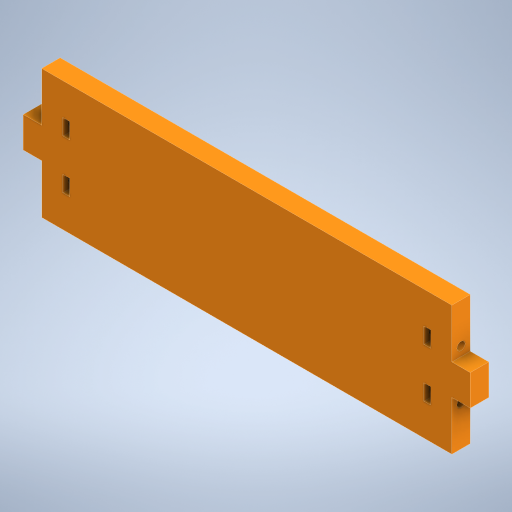
# Autodesk Inventor part: frame_upper3
Saved by Autodesk Inventor 2024 (Build 280153000, 153)
## iProperties
Created: 2024-09-08
Part Number: frame_upper3
Material: 일반
Document SubType Name: Modeling
Designer: jmha0
Density: 1 g/cm^3
Appearance: 주황색
Author: jmha0
Autodesk Inventor part; units mm, degrees
ref_plane "YZ Plane" through (0, 0, 0) normal (1, 0, 0) x (0, 1, 0)
ref_plane "XZ Plane" through (0, 0, 0) normal (0, 1, 0) x (-1, 0, 0)
ref_plane "XY Plane" through (0, 0, 0) normal (0, 0, 1) x (1, 0, 0)
sketch "스케치1" plane through (0, 0, 0) normal (0, 0, 1) x (1, 0, 0)
  line L0 (0, 0) -> (133.5, 0)
  line L1 (133.5, 0) -> (133.5, 42)
  line L2 (133.5, 42) -> (0, 42)
  line L3 (0, 42) -> (0, 0)
  dimension "d0" = 133.5
  dimension "d1" = 42
  constraints: 8 end point, 2 parallel, 1 horizontal, 1 perpendicular
  measures "d0" distance of L2.end L1.end
  measures "d1" distance of L1.end L0.end
extrude "돌출1" add sketch "스케치1" along normal blind 6
sketch "스케치2" plane through (133.5, 0, 0) normal (1, 0, 0) x (0, 0, -1)
  line L0 (0, 0) -> (0, 42) projected
  line L1 (0, 42) -> (-6, 42) projected
  line L2 (-6, 0) -> (-6, 42) projected
  line L3 (0, 0) -> (-6, 0) projected
  line L4 (-6, 16) -> (0, 16)
  line L5 (0, 16) -> (0, 26)
  line L6 (0, 26) -> (-6, 26)
  line L7 (-6, 26) -> (-6, 16)
  line L8 (-6, 16) -> (0, 26) construction
  line L9 (0, 16) -> (-6, 26) construction
  point P0 (-3, 21)
  dimension "d4" = 10
  constraints: 12 end point, 2 midpoint, 2 parallel, 1 horizontal, 1 perpendicular, 1 point on line
  measures "d4" distance of L5.end L4.end
extrude "돌출2" add sketch "스케치2" along normal blind 6 contours L4 L2 L6 L0
sketch "스케치3" plane through (0, 0, 0) normal (-1, 0, 0) x (0, 0, 1)
  line L0 (6, 26) -> (0, 26) projected
  line L1 (0, 16) -> (6, 16) projected
  line L2 (0, 42) -> (0, 0) projected
  line L3 (0, 0) -> (6, 0) projected
  line L4 (6, 42) -> (6, 0) projected
  line L5 (0, 42) -> (6, 42) projected
extrude "돌출3" add sketch "스케치3" along normal blind 6 contours L4 L1 L2 L0
sketch "스케치4" plane through (0, 42, 0) normal (-1, 0, 0) x (0, 0, 1)
  line L0 (0, -16) -> (6, -16) projected
  line L1 (6, 0) -> (6, -16) projected
  line L2 (0, 0) -> (6, 0) projected
  line L3 (0, 0) -> (0, -16) projected
  line L4 (6, -26) -> (0, -26) projected
  line L5 (0, -26) -> (0, -42) projected
  line L6 (0, -42) -> (6, -42) projected
  line L7 (6, -26) -> (6, -42) projected
  line L8 (0, -16) -> (6, -16)
  line L9 (6, -16) -> (6, -10)
  line L10 (6, -10) -> (0, -10)
  line L11 (0, -10) -> (0, -16)
  line L12 (6, -26) -> (0, -26)
  line L13 (0, -26) -> (0, -32)
  line L14 (0, -32) -> (6, -32)
  line L15 (6, -32) -> (6, -26)
  circle A0 centre (3, -13) radius 1.35
  circle A1 centre (3, -29) radius 1.35
  dimension "d9" = 6
  dimension "d10" = 6
  dimension "d11" = 6
  dimension "d12" = 6
  dimension "d13" = 2.7
  dimension "d14" = 2.7
  constraints: 16 end point, 4 parallel, 2 centre point, 2 horizontal, 2 perpendicular
  measures "d9" distance of L10.end L9.end
  measures "d10" distance of L9.end L8.end
  measures "d11" distance of L14.end L13.end
  measures "d12" distance of L13.end L12.end
  measures "d13" diameter of A0
  measures "d14" diameter of A1
extrude "돌출4" cut sketch "스케치4" against normal blind 16 contours A0 | A1
sketch "스케치5" plane through (133.5, 42, 6) normal (1, 0, 0) x (0, 0, -1)
  circle A0 centre (3, -13) radius 1.35 projected
  circle A1 centre (3, -29) radius 1.35 projected
  point P0 (6, -42)
extrude "돌출5" cut sketch "스케치5" against normal blind 16
sketch "스케치7" plane through (0, 0, 0) normal (0, 0, -1) x (-1, 0, 0)
  line L0 (-133.5, 0) -> (-133.5, 16) projected
  line L1 (-133.5, 11.65) -> (-133.5, 14.35) projected
  line L2 (-133.5, 0) -> (-133.5, 16) projected
  line L3 (-133.5, 11.65) -> (-133.5, 14.35) projected
  line L4 (-133.5, 0) -> (-133.5, 16) projected
  line L5 (-133.5, 0) -> (-133.5, 16) projected
  line L6 (-133.5, 42) -> (0, 42) projected
  line L7 (-133.5, 42) -> (0, 42) projected
  line L8 (0, 0) -> (-133.5, 0) projected
  line L9 (0, 0) -> (-133.5, 0) projected
  line L10 (-133.5, 16) -> (-139.5, 16) projected
  line L11 (-133.5, 16) -> (-139.5, 16) projected
  line L12 (-133.5, 16) -> (-139.5, 16) projected
  line L13 (-133.5, 16) -> (-139.5, 16) projected
  line L14 (-117.5, 11.65) -> (-117.5, 14.35) projected
  line L15 (-117.5, 11.65) -> (-117.5, 14.35) projected
  line L16 (-133.5, 11.65) -> (-133.5, 14.35) projected
  line L17 (-117.5, 11.65) -> (-117.5, 14.35) projected
  line L18 (-133.5, 26) -> (-139.5, 26) projected
  line L19 (-133.5, 26) -> (-139.5, 26) projected
  line L20 (-133.5, 26) -> (-139.5, 26) projected
  line L21 (-133.5, 26) -> (-139.5, 26) projected
  line L22 (-139.5, 26) -> (-139.5, 16) projected
  line L23 (-139.5, 16) -> (-139.5, 26) projected
  line L24 (-117.5, 27.65) -> (-117.5, 30.35) projected
  line L25 (-133.5, 27.65) -> (-133.5, 30.35) projected
  line L26 (-133.5, 26) -> (-133.5, 42) projected
  line L27 (-133.5, 26) -> (-133.5, 42) projected
  line L28 (-133.5, 27.65) -> (-133.5, 30.35) projected
  line L29 (-133.5, 26) -> (-133.5, 42) projected
  line L30 (-133.5, 26) -> (-133.5, 42) projected
  line L31 (0, 16) -> (0, 0) projected
  line L32 (0, 16) -> (0, 0) projected
  line L33 (0, 0) -> (-133.5, 0) projected
  line L34 (0, 0) -> (-133.5, 0) projected
  line L35 (-133.5, 0) -> (-133.5, 16) projected
  line L36 (-133.5, 16) -> (-139.5, 16) projected
  line L37 (-139.5, 26) -> (-139.5, 16) projected
  line L38 (-133.5, 26) -> (-139.5, 26) projected
  line L39 (-133.5, 26) -> (-133.5, 42) projected
  line L40 (-133.5, 42) -> (0, 42) projected
  line L41 (0, 42) -> (0, 26) projected
  line L42 (0, 26) -> (6, 26) projected
  line L43 (6, 16) -> (6, 26) projected
  line L44 (0, 16) -> (6, 16) projected
  line L45 (0, 16) -> (0, 0) projected
  line L46 (0, 0) -> (-133.5, 0) projected
  line L47 (-133.5, 0) -> (-133.5, 16) projected
  line L48 (0, 0) -> (-133.5, 0) projected
  line L49 (0, 16) -> (0, 0) projected
  line L50 (0, 16) -> (6, 16) projected
  line L51 (6, 26) -> (6, 16) projected
  line L52 (0, 26) -> (6, 26) projected
  line L53 (0, 42) -> (0, 26) projected
  line L54 (-133.5, 42) -> (0, 42) projected
  line L55 (-133.5, 26) -> (-133.5, 42) projected
  line L56 (-133.5, 26) -> (-139.5, 26) projected
  line L57 (-139.5, 16) -> (-139.5, 26) projected
  line L58 (-133.5, 16) -> (-139.5, 16) projected
  line L59 (0, 42) -> (0, 26) projected
  line L60 (0, 42) -> (0, 26) projected
  line L61 (-133.5, 42) -> (0, 42) projected
  line L62 (-133.5, 42) -> (0, 42) projected
  line L63 (-133.5, 27.65) -> (-133.5, 30.35) projected
  line L64 (-139.5, 26) -> (-139.5, 16) projected
  line L65 (-139.5, 16) -> (-139.5, 26) projected
  line L66 (-16, 14.35) -> (-16, 11.65) projected
  line L67 (-16, 14.35) -> (-16, 11.65) projected
  line L68 (0, 14.35) -> (0, 11.65) projected
  line L69 (0, 16) -> (0, 0) projected
  line L70 (0, 16) -> (0, 0) projected
  line L71 (-16, 30.35) -> (-16, 27.65) projected
  line L72 (0, 30.35) -> (0, 27.65) projected
  line L73 (-16, 14.35) -> (-16, 11.65) projected
  line L74 (0, 14.35) -> (0, 11.65) projected
  line L75 (0, 14.35) -> (0, 11.65) projected
  line L76 (0, 30.35) -> (0, 27.65) projected
  line L77 (0, 30.35) -> (0, 27.65) projected
  line L78 (0, 42) -> (0, 26) projected
  line L79 (0, 42) -> (0, 26) projected
  line L80 (6, 16) -> (6, 26) projected
  line L81 (0, 16) -> (6, 16) projected
  line L82 (6, 26) -> (6, 16) projected
  line L83 (6, 16) -> (6, 26) projected
  line L84 (0, 16) -> (6, 16) projected
  line L85 (0, 16) -> (6, 16) projected
  line L86 (0, 16) -> (6, 16) projected
  line L87 (0, 26) -> (6, 26) projected
  line L88 (0, 26) -> (6, 26) projected
  line L89 (0, 26) -> (6, 26) projected
  line L90 (6, 26) -> (6, 16) projected
  line L91 (-16, 30.35) -> (-16, 27.65) projected
  line L92 (-16, 30.35) -> (-16, 27.65) projected
  line L93 (0, 26) -> (6, 26) projected
  line L94 (-117.5, 27.65) -> (-117.5, 30.35) projected
  line L95 (-117.5, 27.65) -> (-117.5, 30.35) projected
  line L96 (-133.5, 30.35) -> (-117.5, 30.35) projected
  line L97 (-133.5, 27.65) -> (-117.5, 27.65) projected
  line L98 (-133.5, 14.35) -> (-117.5, 14.35) projected
  line L99 (-133.5, 11.65) -> (-117.5, 11.65) projected
  line L100 (0, 30.35) -> (-16, 30.35) projected
  line L101 (0, 27.65) -> (-16, 27.65) projected
  line L102 (0, 14.35) -> (-16, 14.35) projected
  line L103 (0, 11.65) -> (-16, 11.65) projected
  line L104 (-126.6, 26.4) -> (-124.4, 26.4)
  line L105 (-124.4, 26.4) -> (-124.4, 31.6)
  line L106 (-124.4, 31.6) -> (-126.6, 31.6)
  line L107 (-126.6, 31.6) -> (-126.6, 26.4)
  line L108 (-126.6, 26.4) -> (-124.4, 31.6) construction
  line L109 (-124.4, 26.4) -> (-126.6, 31.6) construction
  line L110 (-126.6, 10.4) -> (-124.4, 10.4)
  line L111 (-124.4, 10.4) -> (-124.4, 15.6)
  line L112 (-124.4, 15.6) -> (-126.6, 15.6)
  line L113 (-126.6, 15.6) -> (-126.6, 10.4)
  line L114 (-126.6, 10.4) -> (-124.4, 15.6) construction
  line L115 (-124.4, 10.4) -> (-126.6, 15.6) construction
  line L116 (-9.1, 26.4) -> (-6.9, 26.4)
  line L117 (-6.9, 26.4) -> (-6.9, 31.6)
  line L118 (-6.9, 31.6) -> (-9.1, 31.6)
  line L119 (-9.1, 31.6) -> (-9.1, 26.4)
  line L120 (-9.1, 26.4) -> (-6.9, 31.6) construction
  line L121 (-6.9, 26.4) -> (-9.1, 31.6) construction
  line L122 (-9.1, 10.4) -> (-6.9, 10.4)
  line L123 (-6.9, 10.4) -> (-6.9, 15.6)
  line L124 (-6.9, 15.6) -> (-9.1, 15.6)
  line L125 (-9.1, 15.6) -> (-9.1, 10.4)
  line L126 (-9.1, 10.4) -> (-6.9, 15.6) construction
  line L127 (-6.9, 10.4) -> (-9.1, 15.6) construction
  point P0 (-125.5, 29)
  point P1 (-125.5, 13)
  point P2 (-8, 29)
  point P3 (-8, 13)
  dimension "d27" = 2.2
  dimension "d28" = 5.2
  dimension "d29" = 5.2
  dimension "d30" = 2.2
  dimension "d31" = 5.2
  dimension "d32" = 5.2
  constraints: 48 end point, 8 midpoint, 8 parallel, 4 horizontal, 4 perpendicular, 2 point on line, 5 other
  measures "d27" distance of L106.end L105.end
  measures "d28" distance of L105.end L104.end
  measures "d29" distance of L111.end L110.end
  measures "d30" distance of L118.end L117.end
  measures "d31" distance of L117.end L116.end
  measures "d32" distance of L123.end L122.end
extrude "돌출7" cut sketch "스케치7" against normal blind 16 contours L113 L98 L111 L99 | L99 L111 L110 L113 | L113 L112 L111 L98 | L123 L122 L125 L103 | L103 L125 L102 L123 | L102 L125 L124 L123 | L107 L96 L105 L97 | L97 L105 L104 L107 | L107 L106 L105 L96 | L117 L116 L119 L101 | L101 L119 L100 L117 | L100 L119 L118 L117
sketch "스케치8" plane through (0, 0, 6) normal (0, 0, 1) x (1, 0, 0)
  line L0 (9.1, 26.4) -> (6.9, 26.4) projected
  line L1 (6.9, 26.4) -> (6.9, 31.6) projected
  line L2 (6.9, 31.6) -> (9.1, 31.6) projected
  line L3 (9.1, 31.6) -> (9.1, 26.4) projected
  line L4 (126.6, 10.4) -> (124.4, 10.4) projected
  line L5 (124.4, 10.4) -> (124.4, 15.6) projected
  line L6 (124.4, 15.6) -> (126.6, 15.6) projected
  line L7 (126.6, 15.6) -> (126.6, 10.4) projected
  line L8 (9.1, 10.4) -> (6.9, 10.4) projected
  line L9 (6.9, 10.4) -> (6.9, 15.6) projected
  line L10 (6.9, 15.6) -> (9.1, 15.6) projected
  line L11 (9.1, 15.6) -> (9.1, 10.4) projected
  line L12 (126.6, 26.4) -> (124.4, 26.4) projected
  line L13 (124.4, 26.4) -> (124.4, 31.6) projected
  line L14 (124.4, 31.6) -> (126.6, 31.6) projected
  line L15 (126.6, 31.6) -> (126.6, 26.4) projected
  line L16 (133.5, 0) -> (133.5, 16) projected
  line L17 (133.5, 16) -> (139.5, 16) projected
  line L18 (139.5, 26) -> (139.5, 16) projected
  line L19 (133.5, 26) -> (139.5, 26) projected
  line L20 (133.5, 26) -> (133.5, 42) projected
  line L21 (133.5, 42) -> (0, 42) projected
  line L22 (0, 42) -> (0, 26) projected
  line L23 (0, 26) -> (-6, 26) projected
  line L24 (-6, 16) -> (-6, 26) projected
  line L25 (0, 16) -> (-6, 16) projected
  line L26 (0, 16) -> (0, 0) projected
  line L27 (0, 0) -> (133.5, 0) projected
  line L28 (133.5, 0) -> (0, 0)
  line L29 (0, 0) -> (0, 42)
  line L30 (0, 42) -> (133.5, 42)
  line L31 (133.5, 42) -> (133.5, 0)
  constraints: 8 end point, 2 parallel, 1 horizontal, 1 perpendicular
extrude "돌출8" cut sketch "스케치8" against normal through all contours L31 L19 L18 L17 | L25 L24 L23 L29
sketch "스케치9" plane through (133.5, 0, 0) normal (1, 0, 0) x (0, 0, -1)
  circle A0 centre (-3, 29) radius 1.35 projected
  circle A1 centre (-3, 13) radius 1.35 projected
  line L0 (-6, 0) -> (-6, 42) projected
  line L1 (0, 0) -> (-6, 0) projected
  line L2 (0, 0) -> (0, 42) projected
  line L3 (0, 42) -> (-6, 42) projected
  line L4 (-6, 16) -> (0, 16)
  line L5 (0, 16) -> (0, 26)
  line L6 (0, 26) -> (-6, 26)
  line L7 (-6, 26) -> (-6, 16)
  line L8 (-6, 16) -> (0, 26) construction
  line L9 (0, 16) -> (-6, 26) construction
  point P0 (-3, 21)
  dimension "d37" = 10
  constraints: 12 end point, 2 midpoint, 2 parallel, 1 horizontal, 1 perpendicular, 1 point on line
  measures "d37" distance of L5.end L4.end
extrude "돌출9" add sketch "스케치9" along normal blind 6 contours L0 L6 L2 L4
sketch "스케치10" plane through (0, 0, 0) normal (-1, 0, 0) x (0, 0, 1)
  line L0 (6, 15.6) -> (6, 10.4) projected
  line L1 (6, 10.4) -> (6, 15.6) projected
  line L2 (0, 15.6) -> (0, 10.4) projected
  line L3 (6, 31.6) -> (6, 26.4) projected
  line L4 (0, 26.4) -> (0, 31.6) projected
  line L5 (0, 10.4) -> (0, 15.6) projected
  line L6 (6, 0) -> (6, 16) projected
  line L7 (0, 0) -> (0, 16) projected
  line L8 (0, 0) -> (6, 0) projected
  line L9 (0, 16) -> (6, 16) projected
  line L10 (6, 0) -> (6, 16) projected
  line L11 (0, 0) -> (6, 0) projected
  line L12 (0, 0) -> (0, 16) projected
  circle A0 centre (3, 13) radius 1.35 projected
  line L13 (6, 26) -> (6, 42) projected
  line L14 (0, 42) -> (6, 42) projected
  line L15 (6, 26) -> (0, 26) projected
  line L16 (0, 26) -> (0, 42) projected
  line L17 (0, 42) -> (6, 42) projected
  line L18 (6, 26) -> (6, 42) projected
  circle A1 centre (3, 29) radius 1.35 projected
  line L19 (0, 26) -> (0, 42) projected
  line L20 (0, 31.6) -> (0, 26.4) projected
  line L21 (6, 26.4) -> (6, 31.6) projected
  line L22 (6, 31.6) -> (6, 26.4) projected
  line L23 (6, 26.4) -> (6, 31.6) projected
  circle A2 centre (3, 29) radius 1.35 projected
  circle A3 centre (3, 29) radius 1.35 projected
  circle A4 centre (3, 13) radius 1.35 projected
  circle A5 centre (3, 13) radius 1.35 projected
  circle A6 centre (3, 29) radius 1.35 projected
  line L24 (0, 31.6) -> (6, 31.6) projected
  line L25 (0, 26.4) -> (6, 26.4) projected
  line L26 (6, 31.6) -> (6, 26.4) projected
  line L27 (0, 31.6) -> (6, 31.6) projected
  line L28 (0, 26.4) -> (0, 31.6) projected
  line L29 (0, 26.4) -> (6, 26.4) projected
  circle A7 centre (3, 29) radius 1.35 projected
  circle A8 centre (3, 29) radius 1.35 projected
  circle A9 centre (3, 29) radius 1.35 projected
  circle A10 centre (3, 13) radius 1.35 projected
  circle A11 centre (3, 13) radius 1.35 projected
  line L30 (0, 31.6) -> (6, 31.6) projected
  line L31 (0, 31.6) -> (6, 31.6) projected
  line L32 (0, 31.6) -> (6, 31.6) projected
  circle A12 centre (3, 29) radius 1.35 projected
  line L33 (0, 26.4) -> (6, 26.4) projected
  line L34 (6, 26.4) -> (6, 31.6) projected
  line L35 (0, 26.4) -> (6, 26.4) projected
  line L36 (0, 31.6) -> (0, 26.4) projected
  line L37 (0, 31.6) -> (6, 31.6) projected
  circle A13 centre (3, 29) radius 1.35 projected
  line L38 (0, 26.4) -> (6, 26.4) projected
  line L39 (0, 26.4) -> (6, 26.4) projected
  line L40 (0, 31.6) -> (0, 26.4) projected
  line L41 (0, 26.4) -> (0, 31.6) projected
  line L42 (6, 15.6) -> (6, 10.4) projected
  line L43 (0, 42) -> (6, 42) projected
  line L44 (0, 42) -> (6, 42) projected
  line L45 (6, 0) -> (6, 16) projected
  line L46 (6, 26) -> (6, 16) projected
  line L47 (6, 26) -> (6, 42) projected
  line L48 (6, 42) -> (6, 0) projected
  line L49 (6, 26.4) -> (6, 31.6) projected
  line L50 (6, 31.6) -> (6, 26.4) projected
  line L51 (6, 10.4) -> (6, 15.6) projected
  line L52 (6, 15.6) -> (6, 10.4) projected
  line L53 (6, 10.4) -> (6, 15.6) projected
  line L54 (6, 15.6) -> (6, 10.4) projected
  line L55 (6, 26.4) -> (6, 31.6) projected
  line L56 (6, 31.6) -> (6, 26.4) projected
  line L57 (0, 0) -> (0, 16) projected
  line L58 (0, 42) -> (0, 0) projected
  line L59 (0, 26) -> (0, 42) projected
  line L60 (0, 16) -> (0, 26) projected
  line L61 (0, 26.4) -> (0, 31.6) projected
  line L62 (0, 31.6) -> (0, 26.4) projected
  line L63 (0, 10.4) -> (0, 15.6) projected
  line L64 (0, 15.6) -> (0, 10.4) projected
  line L65 (0, 10.4) -> (0, 15.6) projected
  line L66 (0, 15.6) -> (0, 10.4) projected
  line L67 (0, 26.4) -> (0, 31.6) projected
  line L68 (0, 31.6) -> (0, 26.4) projected
  line L69 (0, 0) -> (6, 0) projected
  line L70 (0, 0) -> (6, 0) projected
  line L71 (0, 10.4) -> (0, 15.6) projected
  line L72 (0, 15.6) -> (0, 10.4) projected
  line L73 (6, 10.4) -> (6, 15.6) projected
  line L74 (6, 42) -> (6, 0) projected
  circle A14 centre (3, 29) radius 1.35 projected
  circle A15 centre (3, 13) radius 1.35 projected
  line L75 (0, 16) -> (0, 26) projected
  line L76 (6, 26) -> (6, 16) projected
  line L77 (6, 16) -> (0, 16) projected
  line L78 (0, 16) -> (6, 16) projected
  line L79 (0, 26) -> (6, 26) projected
  line L80 (6, 26) -> (0, 26) projected
  line L81 (6, 26) -> (6, 16) projected
  line L82 (6, 16) -> (0, 16) projected
  line L83 (0, 16) -> (0, 26) projected
  line L84 (0, 26) -> (6, 26) projected
  line L85 (0, 16) -> (6, 16) projected
  line L86 (6, 16) -> (0, 16) projected
  line L87 (6, 26) -> (0, 26) projected
  line L88 (0, 26) -> (6, 26) projected
  circle A16 centre (3, 29) radius 1.35 projected
  line L89 (0, 31.6) -> (6, 31.6) projected
  line L90 (0, 31.6) -> (6, 31.6) projected
  circle A17 centre (3, 29) radius 1.35 projected
  line L91 (0, 26.4) -> (6, 26.4) projected
  line L92 (0, 15.6) -> (6, 15.6) projected
  line L93 (0, 26.4) -> (6, 26.4) projected
  circle A18 centre (3, 13) radius 1.35 projected
  circle A19 centre (3, 13) radius 1.35 projected
  line L94 (0, 15.6) -> (6, 15.6) projected
  line L95 (0, 10.4) -> (6, 10.4) projected
  line L96 (0, 10.4) -> (6, 10.4) projected
  circle A20 centre (3, 13) radius 1.35 projected
  line L97 (0, 15.6) -> (6, 15.6) projected
  line L98 (0, 15.6) -> (6, 15.6) projected
  circle A21 centre (3, 13) radius 1.35 projected
  line L99 (0, 10.4) -> (6, 10.4) projected
  line L100 (0, 10.4) -> (6, 10.4) projected
  line L101 (6, 10.4) -> (6, 15.6) projected
  line L102 (0, 10.4) -> (6, 10.4) projected
  line L103 (0, 15.6) -> (0, 10.4) projected
  line L104 (0, 15.6) -> (6, 15.6) projected
  circle A22 centre (3, 13) radius 1.35 projected
  line L105 (0, 15.6) -> (6, 15.6) projected
  line L106 (0, 15.6) -> (6, 15.6) projected
  line L107 (6, 15.6) -> (6, 10.4) projected
  line L108 (0, 15.6) -> (6, 15.6) projected
  line L109 (0, 10.4) -> (0, 15.6) projected
  line L110 (0, 10.4) -> (6, 10.4) projected
  circle A23 centre (3, 13) radius 1.35 projected
  line L111 (0, 0) -> (6, 0) projected
  line L112 (0, 42) -> (0, 0) projected
  circle A24 centre (3, 13) radius 1.35 projected
  circle A25 centre (3, 29) radius 1.35 projected
  line L113 (6, 42) -> (6, 0) projected
  line L114 (0, 42) -> (6, 42) projected
  line L115 (0, 42) -> (0, 0) projected
  line L116 (0, 0) -> (6, 0) projected
  circle A26 centre (3, 13) radius 1.35 projected
  circle A27 centre (3, 29) radius 1.35 projected
  circle A28 centre (3, 13) radius 1.35 projected
  circle A29 centre (3, 13) radius 1.35 projected
  circle A30 centre (3, 13) radius 1.35 projected
  line L117 (0, 42) -> (6, 42) projected
  circle A31 centre (3, 29) radius 1.35 projected
  circle A32 centre (3, 29) radius 1.35 projected
  circle A33 centre (3, 29) radius 1.35 projected
  circle A34 centre (3, 13) radius 1.35 projected
  circle A35 centre (3, 29) radius 1.35 projected
  circle A36 centre (3, 13) radius 1.35 projected
  circle A37 centre (3, 13) radius 1.35 projected
  circle A38 centre (3, 29) radius 1.35 projected
  circle A39 centre (3, 29) radius 1.35 projected
  line L118 (6, 10.4) -> (6, 15.6) projected
  line L119 (0, 10.4) -> (6, 10.4) projected
  line L120 (0, 15.6) -> (0, 10.4) projected
  line L121 (0, 15.6) -> (6, 15.6) projected
  circle A40 centre (3, 13) radius 1.35 projected
  line L122 (6, 26.4) -> (6, 31.6) projected
  line L123 (0, 26.4) -> (6, 26.4) projected
  line L124 (0, 31.6) -> (0, 26.4) projected
  line L125 (0, 31.6) -> (6, 31.6) projected
  circle A41 centre (3, 29) radius 1.35 projected
  line L126 (0, 10.4) -> (6, 10.4) projected
  line L127 (0, 10.4) -> (6, 10.4) projected
  line L128 (0, 15.6) -> (6, 15.6) projected
  line L129 (0, 15.6) -> (6, 15.6) projected
  line L130 (0, 26.4) -> (6, 26.4) projected
  line L131 (0, 26.4) -> (6, 26.4) projected
  line L132 (0, 31.6) -> (6, 31.6) projected
  line L133 (0, 31.6) -> (6, 31.6) projected
  line L134 (6, 15.6) -> (6, 10.4) projected
  line L135 (0, 15.6) -> (6, 15.6) projected
  line L136 (0, 10.4) -> (0, 15.6) projected
  line L137 (0, 10.4) -> (6, 10.4) projected
  circle A42 centre (3, 13) radius 1.35 projected
  circle A43 centre (3, 29) radius 1.35 projected
  circle A44 centre (3, 29) radius 1.35 projected
  circle A45 centre (3, 13) radius 1.35 projected
  circle A46 centre (3, 13) radius 1.35 projected
  line L138 (6, 31.6) -> (6, 26.4) projected
  line L139 (0, 31.6) -> (6, 31.6) projected
  line L140 (0, 26.4) -> (0, 31.6) projected
  line L141 (0, 26.4) -> (6, 26.4) projected
  circle A47 centre (3, 29) radius 1.35 projected
  line L142 (0, 10.4) -> (6, 10.4) projected
  line L143 (0, 10.4) -> (6, 10.4) projected
  constraints: 21 other
extrude "돌출10" add sketch "스케치10" along normal blind 6 contours L9 L58 L15 L46
